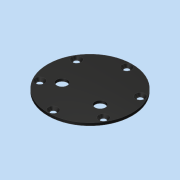
# Autodesk Inventor part: foreHullInsert
Saved by Autodesk Inventor 2017 (Build 210142000, 142)
## iProperties
Created: 2016-09-09
Part Number: foreHullInsert
Material: Generic
Document SubType Name: Modeling
Designer: techn
Density: 1 g/cm^3
Appearance: Glossy - Black
Mass: 764.223 g
Surface Area: 456.432 cm^2
Volume: 764.223 cm^3
Author: techn
Autodesk Inventor part; units mm, degrees
ref_plane "YZ Plane" through (0, 0, 0) normal (1, 0, 0) x (0, 1, 0)
ref_plane "XZ Plane" through (0, 0, 0) normal (0, 1, 0) x (-1, 0, 0)
ref_plane "XY Plane" through (0, 0, 0) normal (0, 0, 1) x (1, 0, 0)
sketch "Sketch6" plane through (0, 0, 0) normal (0, 0, 1) x (1, 0, 0)
  line L0 (540.6478, 1219.1491) -> (540.6478, -58.7076) construction
  line L1 (540.6478, -58.7076) -> (-407.4394, -58.7076) construction
  line L2 (-407.4394, -58.7076) -> (-407.4394, 1219.1491) construction
  line L3 (-407.4394, 1219.1491) -> (540.6478, 1219.1491) construction
  point P0 (0, 0)
  constraints: 2 other
sketch "Sketch5" plane through (0, 0, 0) normal (0, 0, 1) x (1, 0, 0)
  line L0 (0, 0) -> (0, 142.24)
  line L1 (0, 142.24) -> (50.8, 142.24)
  line L2 (50.8, 142.24) -> (-50.8, 142.24)
  line L3 (50.8, 142.24) -> (45.2986, 0) construction
  line L4 (45.2986, 0) -> (0, 0) construction
  spline S0 degree 2 poles (50.8, 142.24) (45.2986, 0) (0, 0) knots 1 1 1 2 2 2
  line L5 (-50.8, 142.24) -> (-45.2986, 0) construction
  line L6 (-45.2986, 0) -> (0, 0) construction
  spline S1 degree 2 poles (-50.8, 142.24) (-45.2986, 0) (0, 0) knots 1 1 1 2 2 2
  dimension "d20" = 142.24
  dimension "d21" = 50.8
  dimension "d22" = 101.6
  constraints: 6 end point, 1 horizontal, 1 perpendicular, 1 point on line, 1 symmetric about line, 1 vertical, 6 other
  measures "d20" distance of L0.start L0.end
  measures "d21" distance of L0.end L1.end
  measures "d22" distance of L1.end L2.end
revolve "Revolution1" add sketch "Sketch5" angle 360 about axis through (0, 0, 0) along (0, 1, 0) contours L0 L1 S0
ref_plane "Work Plane1" through (0, 21.59, 0) normal (0, 1, 0) x (1, 0, 0)
sketch "Sketch9" plane through (0, 21.59, 0) normal (0, 1, 0) x (1, 0, 0)
  line L0 (-101.4531, 67.0538) -> (104.6936, 67.0538)
  line L1 (104.6936, 67.0538) -> (104.6936, -70.5436)
  line L2 (104.6936, -70.5436) -> (-101.4531, -70.5436)
  line L3 (-101.4531, -70.5436) -> (-101.4531, 67.0538)
  point P0 (0, 0)
  constraints: 8 end point, 2 parallel, 1 horizontal, 1 perpendicular
extrude "Extrusion2" cut sketch "Sketch9" along normal through all
sketch "Sketch10" plane through (0, 21.59, 0) normal (0, 1, 0) x (1, 0, 0)
  circle A0 centre (0, 0) radius 29.2557
  circle A1 centre (0, 0) radius 25.4
  dimension "d75" = 58.5114
  dimension "d76" = 50.8
  constraints: 2 centre point, 2 coincident, 1 other
  measures "d75" diameter of A0
  measures "d76" diameter of A1
extrude "Extrusion3" add sketch "Sketch10" along normal blind 1.5875 contours A1
extrude "Extrusion4" cut sketch "Sketch10" against normal through all contours A0 | A1
sketch "Sketch11" plane through (0, 23.1775, 0) normal (0, 1, 0) x (1, 0, 0)
  line L0 (0, 0) -> (0, 22.225)
  circle A0 centre (0, 22.225) radius 1.5875
  circle A1 centre (-19.2474, 11.1125) radius 1.5875
  circle A2 centre (-19.2474, -11.1125) radius 1.5875
  circle A3 centre (0, -22.225) radius 1.5875
  circle A4 centre (19.2474, -11.1125) radius 1.5875
  circle A5 centre (19.2474, 11.1125) radius 1.5875
  dimension "d81" = 22.225
  dimension "d82" = 3.175
  dimension "d85" = 360
  constraints: 6 centre point, 2 end point, 1 coincident, 1 vertical, 13 other
  measures "d81" distance of L0.start L0.end
  measures "d82" diameter of A0
extrude "Extrusion5" cut sketch "Sketch11" against normal blind 1.5875
chamfer "Chamfer1" distance 1.27 angle 45 6 edges at (17.6599, 23.1775, 11.1125) (17.6599, 23.1775, -11.1125) (-1.5875, 23.1775, -22.225) (-20.8349, 23.1775, -11.1125) (-20.8349, 23.1775, 11.1125) (-1.5875, 23.1775, 22.225)
sketch "Sketch12" plane through (0, 23.1775, 0) normal (0, 1, 0) x (1, 0, 0)
  line L0 (0, 0) -> (11.5101, -5.3673)
  line L1 (0, 0) -> (12.7, 0) construction
  circle A0 centre (11.5101, -5.3673) radius 3.175
  circle A1 centre (-11.5101, -5.3673) radius 3.175
  line L2 (0, 0) -> (-11.5101, -5.3673) construction
  dimension "d92" = 12.7
  dimension "d93" = 25
  dimension "d94" = 6.35
  dimension "d95" = 6.35
  constraints: 6 end point, 2 centre point, 2 equal length, 1 coincident, 1 horizontal, 1 horizontal alignment
  measures "d92" distance of L0.start L0.end
  measures "d93" angle of L0 L1
  measures "d94" diameter of A0
  measures "d95" diameter of A1
extrude "Extrusion6" cut sketch "Sketch12" against normal through all
body "Solid1"
